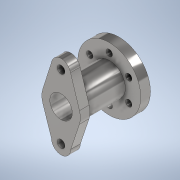
# Autodesk Inventor part: PIEZA_3D_2EX
Saved by Autodesk Inventor 2021 (Build 250183000, 183)
## iProperties
Created: 2021-02-09
Part Number: PIEZA_3D_2EX
Material: Generic
Document SubType Name: Modeling
Designer: aby_2
Density: 1 g/cm^3
Appearance: Steel - Polished
Author: aby_2
Autodesk Inventor part; units mm, degrees
ref_plane "YZ Plane" through (0, 0, 0) normal (1, 0, 0) x (0, 1, 0)
ref_plane "XZ Plane" through (0, 0, 0) normal (0, 1, 0) x (-1, 0, 0)
ref_plane "XY Plane" through (0, 0, 0) normal (0, 0, 1) x (1, 0, 0)
sketch "Sketch1" plane through (0, 0, 0) normal (0, 0, 1) x (1, 0, 0)
  circle A0 centre (0, 0) radius 49
  dimension "d0" = 98
  constraints: 1 centre point, 1 coincident
  measures "d0" diameter of A0
extrude "Extrusion1" add sketch "Sketch1" along normal blind 15
sketch "Sketch2" plane through (0, 0, 15) normal (0, 0, 1) x (1, 0, 0)
  circle A0 centre (0, 0) radius 35
  circle A1 centre (0, 35) radius 5
  circle A2 centre (-30.3109, 17.5) radius 5
  circle A3 centre (-30.3109, -17.5) radius 5
  circle A4 centre (0, -35) radius 5
  circle A5 centre (30.3109, -17.5) radius 5
  circle A6 centre (30.3109, 17.5) radius 5
  dimension "d3" = 70
  dimension "d4" = 10
  dimension "d7" = 360
  constraints: 6 centre point, 1 coincident, 1 vertical alignment, 15 other
  measures "d4" diameter of A1
extrude "Extrusion2" cut sketch "Sketch2" against normal up to next contours A6 A0 | A0 A6 | A5 A0 | A0 A5 | A1 A0 | A0 A1 | A4 A0 | A0 A4 | A2 A0 | A0 A2 | A3 A0 | A0 A3
sketch "Sketch3" plane through (0, 0, 15) normal (0, 0, 1) x (1, 0, 0)
  circle A0 centre (0, 0) radius 25
  dimension "d11" = 50
  constraints: 1 centre point, 1 coincident
  measures "d11" diameter of A0
extrude "Extrusion3" add sketch "Sketch3" along normal blind 75
sketch "Sketch4" plane through (0, 0, 15) normal (0, 0, 1) x (1, 0, 0)
  circle A0 centre (0, 0) radius 13
  dimension "d14" = 26
  constraints: 1 centre point, 1 coincident
  measures "d14" diameter of A0
extrude "Extrusion4" cut sketch "Sketch4" along normal blind 45
sketch "Sketch5" plane through (0, 0, 90) normal (0, 0, 1) x (1, 0, 0)
  line L0 (0, 0) -> (0, 50)
  line L1 (0, 0) -> (0, -50)
  arc A0 (-14.6459, -46.76) -> (14.6459, -46.76) centre (0, -50) ccw
  arc A1 (14.6459, 46.76) -> (-14.6459, 46.76) centre (0, 50) ccw
  circle A2 centre (0, 0) radius 49 projected
  circle A3 centre (0, 50) radius 6
  circle A4 centre (0, -50) radius 6
  line L2 (-15, -50) -> (-28.4697, -9.4591)
  line L3 (15, -50) -> (28.4697, -9.4591)
  line L4 (-14.6459, 53.24) -> (-28.6072, 9.035)
  line L5 (14.6459, 53.24) -> (28.6072, 9.035)
  arc A5 (-28.6072, 9.035) -> (-28.4697, -9.4591) centre (0, 0) ccw
  arc A6 (28.4697, -9.4591) -> (28.6072, 9.035) centre (0, 0) ccw
  point P0 (16.254, -46.2256)
  point P1 (16.9391, 45.979)
  point P2 (-16.9391, 45.979)
  point P3 (-16.254, -46.2256)
  dimension "d17" = 50
  dimension "d18" = 50
  dimension "d19" = 30
  dimension "d20" = 30
  dimension "d22" = 12
  dimension "d23" = 12
  constraints: 16 point on circle, 12 end point, 6 centre point, 5 coincident, 4 tangent, 2 vertical
  measures "d17" distance of L0.start L0.end
  measures "d18" distance of L0.start L1.end
  measures "d19" diameter of A0
  measures "d20" diameter of A1
  measures "d22" diameter of A3
  measures "d23" diameter of A4
extrude "Extrusion5" add sketch "Sketch5" against normal blind 15 contours L1 A4 A2 L2 A5 L4 A3 L0 | L0 A3 A2 L5 A6 L3 A4 L1 | A2 A1 A3 | A2 A0 A4 | A2 L4 A1 | A1 L5 A2 | A2 L3 A0 | A0 L2 A2
sketch "Sketch6" plane through (0, 0, 90) normal (0, 0, 1) x (1, 0, 0)
  line L0 (15, -50) -> (28.4697, -9.4591) projected
  arc A0 (28.4697, -9.4591) -> (28.6072, 9.035) centre (0, 0) ccw projected
  line L1 (28.6072, 9.035) -> (14.6459, 53.24) projected
  arc A1 (14.6459, 53.24) -> (-14.6459, 53.24) centre (0, 50) ccw projected
  line L2 (-14.6459, 53.24) -> (-28.6072, 9.035) projected
  arc A2 (-28.6072, 9.035) -> (-28.4697, -9.4591) centre (0, 0) ccw projected
  line L3 (-28.4697, -9.4591) -> (-15, -50) projected
  arc A3 (-15, -50) -> (15, -50) centre (0, -50) ccw projected
  circle A4 centre (0, -50) radius 6 projected
  circle A5 centre (0, 50) radius 6 projected
  circle A6 centre (0, 0) radius 17.5
  dimension "d26" = 35
  constraints: 1 centre point
  measures "d26" diameter of A6
extrude "Extrusion6" cut sketch "Sketch6" against normal blind 30 contours A6
body "Solid1"
